Autodesk Fusion 360 part; units mm, degrees
(part 2 of 2)
sketch "Sketch26" plane through (0, 0, -29.65) normal (0, 0, 1) x (-1, 0, 0)
  circle A0 centre (-271.74, -5) radius 4.5
  circle A1 centre (-155, -82.8) radius 4.5
  circle A2 centre (-271.74, -82.8) radius 4.5
  circle A3 centre (-155, -5) radius 4.5
  line L0 (-186.5, -86) -> (-186.5, -90)
  line L1 (-186.5, -90) -> (-147, -90)
  line L2 (-147, -90) -> (-147, 7)
  line L3 (-147, 7) -> (-282, 7)
  line L4 (-282, 7) -> (-282, -90)
  line L5 (-282, -90) -> (-233, -90)
  line L6 (-233, -90) -> (-233, -86)
  line L7 (-233, -86) -> (-186.5, -86)
  line L8 (-243, -90) -> (-263, -90)
  line L9 (-263, -90) -> (-263, -72)
  line L10 (-263, -72) -> (-243, -72)
  line L11 (-243, -72) -> (-243, -90)
  dimension "d246" = 20
  dimension "d247" = 10
  dimension "d248" = 18
  constraint horizontal L8
  constraint vertical L9
  constraint horizontal L10
  constraint vertical L11
  constraint coincident L5 L8.start
  measures "d246" distance of L9 L11
  measures "d247" distance of L6 L11
  measures "d248" distance of L8.end L9.end
extrude "Extrude25" add sketch "Sketch26" along normal blind 5 contours L5 L8 L9 L10 L11 bodies 34
sketch "Sketch27" plane through (0, 0, -24.65) normal (0, 0, 1) x (-1, 0, 0)
  line L0 (-243, -72) -> (-263, -72)
  line L1 (-263, -72) -> (-263, -90)
  line L2 (-263, -90) -> (-243, -90)
  line L3 (-243, -90) -> (-243, -72)
  line L4 (-243, -90) -> (-243.9, -90)
  line L5 (-243.9, -90) -> (-243.9, -72)
  line L6 (-243.9, -72) -> (-243, -72)
  line L7 (-243, -72) -> (-243, -90)
  line L8 (-243.9, -72) -> (-263, -72)
  line L9 (-263, -72) -> (-263, -72.9)
  line L10 (-263, -72.9) -> (-243.9, -72.9)
  line L11 (-243.9, -72.9) -> (-243.9, -72)
  line L12 (-263, -72.9) -> (-262.1, -72.9)
  line L13 (-262.1, -72.9) -> (-262.1, -90)
  line L14 (-262.1, -90) -> (-263, -90)
  line L15 (-263, -90) -> (-263, -72.9)
  dimension "d251" = 0.9
  dimension "d252" = 0.9
  dimension "d253" = 0.9
  constraint horizontal L4
  constraint vertical L5
  constraint horizontal L6
  constraint vertical L7
  constraint coincident L0 L5.end
  constraint coincident L2.end L3.start
  constraint horizontal L8
  constraint vertical L9
  constraint horizontal L10
  constraint vertical L11
  constraint coincident L1 L9.end
  constraint horizontal L12
  constraint vertical L13
  constraint horizontal L14
  constraint vertical L15
  constraint coincident L2 L13.end
  measures "d251" distance of L8 L10
  measures "d252" distance of L5 L7
  measures "d253" distance of L13 L15
extrude "Extrude26" add sketch "Sketch27" along normal blind 1 contours L0 L2 L3 L4 L5 L6 L7 L11 | L0 L1 L5 L8 L9 L10 L11 L12 | L1 L2 L10 L12 L13 L14 L15 bodies 34
sketch "Sketch29" plane through (0, 90, 0) normal (0, -1, 0) x (1, 0, 0)
  line L0 (243, -29.65) -> (243, -23.65)
  line L1 (243, -23.65) -> (243.9, -23.65)
  line L2 (243.9, -23.65) -> (243.9, -24.65)
  line L3 (243.9, -24.65) -> (262.1, -24.65)
  line L4 (262.1, -24.65) -> (262.1, -23.65)
  line L5 (262.1, -23.65) -> (263, -23.65)
  line L6 (263, -23.65) -> (263, -29.65)
  line L7 (263, -29.65) -> (282, -29.65)
  line L8 (282, -29.65) -> (282, -12.65)
  line L9 (282, -12.65) -> (233, -12.65)
  line L10 (233, -12.65) -> (233, -29.65)
  line L11 (233, -29.65) -> (243, -29.65)
  line L12 (248.95, -21) -> (257.3, -21)
  line L13 (257.3, -21) -> (257.3, -25.6)
  line L14 (257.3, -25.6) -> (248.95, -25.6)
  line L15 (248.95, -25.6) -> (248.95, -21)
  dimension "d256" = 5.05
  dimension "d257" = 8.35
  dimension "d258" = 4.6
  dimension "d259" = 3.65
  constraint horizontal L12
  constraint vertical L13
  constraint horizontal L14
  constraint vertical L15
  measures "d256" horizontal distance of L2.end L14.end
  measures "d257" distance of L12.start L12.end
  measures "d258" distance of L12.end L13.end
  measures "d259" distance of L3 L12
extrude "Extrude27" cut sketch "Sketch29" along normal blind -3 and the other way blind -3 contours L3 L12 L13 L15 | L3 L13 L14 L15 bodies 34
sketch "Sketch30" plane through (0, 0, -24.65) normal (0, 0, 1) x (-1, 0, 0)
  line L0 (-248.95, -87) -> (-248.95, -90)
  line L1 (-248.95, -90) -> (-243.9, -90)
  line L2 (-243.9, -90) -> (-243.9, -72.9)
  line L3 (-243.9, -72.9) -> (-262.1, -72.9)
  line L4 (-262.1, -72.9) -> (-262.1, -90)
  line L5 (-262.1, -90) -> (-257.3, -90)
  line L6 (-257.3, -90) -> (-257.3, -87)
  line L7 (-257.3, -87) -> (-248.95, -87)
  circle A0 centre (-247.95, -79.45) radius 1
  circle A1 centre (-258.05, -79.45) radius 1
  dimension "d264" = 4.05
  dimension "d265" = 4.05
  dimension "d266" = 6.55
  dimension "d267" = 6.55
  dimension "d268" = 2
  dimension "d269" = 2
  measures "d264" distance of L2 A0.centre
  measures "d265" distance of L4 A1.centre
  measures "d266" distance of L3 A1.centre
  measures "d267" distance of L3 A0.centre
  measures "d268" diameter of A0
  measures "d269" diameter of A1
extrude "Extrude28" cut sketch "Sketch30" against normal blind 5 contours A0 | A1 bodies 34
sketch "Sketch32" plane through (0, 0, -10) normal (0, 0, 1) x (-1, 0, 0)
  line L0 (-155, -1.5359) -> (-152, -3.2679)
  line L1 (-152, -3.2679) -> (-152, -6.7321)
  line L2 (-152, -6.7321) -> (-155, -8.4641)
  line L3 (-155, -8.4641) -> (-158, -6.7321)
  line L4 (-158, -6.7321) -> (-158, -3.2679)
  line L5 (-158, -3.2679) -> (-155, -1.5359)
  circle A0 centre (-155, -5) radius 4.5
  circle A1 centre (-155, -5) radius 2
  circle A2 centre (-155, -82.8) radius 2
  circle A3 centre (-271.74, -82.8) radius 2
  circle A4 centre (-271.74, -5) radius 2
  circle A5 centre (-271.74, -5) radius 4.5
  circle A6 centre (-271.74, -82.8) radius 4.5
  circle A7 centre (-155, -82.8) radius 4.5
  dimension "d272" = 4
  dimension "d273" = 4
  dimension "d274" = 4
  dimension "d275" = 4
  constraint concentric A0 A1
  constraint concentric A4 A5
  constraint concentric A3 A6
  constraint concentric A2 A7
  measures "d272" diameter of A1
  measures "d273" diameter of A2
  measures "d274" diameter of A3
  measures "d275" diameter of A4
extrude "Extrude29" cut sketch "Sketch32" against normal through all contours A1 | A2 | A3 | A4 bodies 34
sketch "Sketch33" plane through (0, 0, -32.65) normal (0, 0, -1) x (1, 0, 0)
  circle A0 centre (155, -5) radius 2
  circle A1 centre (271.74, -5) radius 2
  circle A2 centre (155, -82.8) radius 2
  circle A3 centre (271.74, -82.8) radius 2
  line L0 (290, -83) -> (285, -83)
  line L1 (285, -83) -> (285, 42)
  line L2 (285, 42) -> (290, 42)
  line L3 (290, 42) -> (290, -83)
  line L4 (295, -88) -> (295, 47)
  arc A4 (295, 47) -> (290, 52) centre (290, 47) ccw
  line L5 (290, 52) -> (139, 52)
  arc A5 (139, 52) -> (134, 47) centre (139, 47) ccw
  line L6 (134, 47) -> (134, -88)
  arc A6 (134, -88) -> (139, -93) centre (139, -88) ccw
  line L7 (139, -93) -> (290, -93)
  arc A7 (290, -93) -> (295, -88) centre (290, -88) ccw
  line L8 (139, -83) -> (139, 42)
  line L9 (139, 42) -> (144, 42)
  line L10 (144, 42) -> (144, -83)
  line L11 (144, -83) -> (139, -83)
  circle A8 centre (155, -5) radius 4.5
  circle A9 centre (271.74, -5) radius 4.5
  circle A10 centre (155, -82.8) radius 4.5
  circle A11 centre (271.74, -82.8) radius 4.5
  dimension "d277" = 9
  dimension "d278" = 9
  dimension "d279" = 9
  dimension "d280" = 9
  constraint concentric A0 A8
  constraint concentric A1 A9
  constraint concentric A2 A10
  constraint concentric A3 A11
  measures "d277" diameter of A8
  measures "d278" diameter of A9
  measures "d279" diameter of A10
  measures "d280" diameter of A11
extrude "Extrude30" cut sketch "Sketch33" against normal blind 1 contours A8 | A9 | A10 | A11 bodies 34
move_body "Move19" bodies 36 to x (1, 0, 0) y (0, 1, 0) z (0, 0, 1) at (0, 57, 0)
move_body "Move20" bodies 36 to x (1, 0, 0) y (0, 1, 0) z (0, 0, 1) at (0.2606, 11.9381, -1)
combine "Combine1" operation add target body 35 tool bodies 36
move_body "Move21" bodies 34 to x (1, 0, 0) y (0, 1, 0) z (0, 0, 1) at (-170, 0, 0)
sketch "Sketch34" plane through (0, -52, 0) normal (0, -1, 0) x (1, 0, 0)
  line L0 (115, 16.35) -> (-26, 16.35)
  line L1 (-26, 16.35) -> (-26, 6.35)
  line L2 (-26, 6.35) -> (-31, 6.35)
  line L3 (-31, 6.35) -> (-31, -12.65)
  line L4 (-31, -12.65) -> (120, -12.65)
  line L5 (120, -12.65) -> (120, 6.35)
  line L6 (120, 6.35) -> (115, 6.35)
  line L7 (115, 6.35) -> (115, 16.35)
  circle A0 centre (105.1711, 6.35) radius 6
  circle A1 centre (105.1711, -21.65) radius 6
  line L8 (120, -32.65) -> (-31, -32.65)
  dimension "d286" = 12
  dimension "d287" = 10
  dimension "d288" = 12
  dimension "d289" = 11
  constraint vertical A0.centre A1.centre
  measures "d286" diameter of A0
  measures "d287" distance of L0 A0.centre
  measures "d288" diameter of A1
  measures "d289" distance of A1.centre L8
extrude "Extrude31" cut sketch "Sketch34" against normal blind 3 contours A1 bodies 34
extrude "Extrude32" cut sketch "Sketch34" against normal blind 3 contours A0 bodies 35
sketch "Sketch35" plane through (0, -7, 0) normal (0, 1, 0) x (-1, 0, 0)
  line L0 (-112, -12.65) -> (23, -12.65)
  line L1 (23, -12.65) -> (23, 13.35)
  line L2 (23, 13.35) -> (-112, 13.35)
  line L3 (-112, 13.35) -> (-112, -12.65)
  line L4 (-102, 6.35) -> (-37, 6.35)
  line L5 (-37, 6.35) -> (-37, -21.65)
  line L6 (-37, -21.65) -> (-102, -21.65)
  line L7 (-102, -21.65) -> (-102, 6.35)
  line L8 (23, -29.65) -> (-112, -29.65)
  dimension "d294" = 8
  dimension "d295" = 7
  dimension "d296" = 10
  dimension "d297" = 60
  dimension "d298" = 43
  constraint horizontal L4
  constraint vertical L5
  constraint horizontal L6
  constraint vertical L7
  measures "d294" distance of L6 L8
  measures "d295" distance of L2 L4
  measures "d296" distance of L3 L7
  measures "d297" distance of L1 L5
  measures "d298" distance of L2 L8
extrude "Extrude33" cut sketch "Sketch35" against normal blind 3 contours L0 L4 L5 L7 | L0 L5 L6 L7 bodies 34 35
sketch "Sketch36" plane through (0, 0, -10) normal (0, 0, 1) x (-1, 0, 0)
  line L0 (-101.74, -1.5359) -> (-98.74, -3.2679)
  line L1 (-98.74, -3.2679) -> (-98.74, -6.7321)
  line L2 (-98.74, -6.7321) -> (-101.74, -8.4641)
  line L3 (-101.74, -8.4641) -> (-104.74, -6.7321)
  line L4 (-104.74, -6.7321) -> (-104.74, -3.2679)
  line L5 (-104.74, -3.2679) -> (-101.74, -1.5359)
  circle A0 centre (-101.74, -5) radius 4.5
  line L6 (-101.74, -5) -> (-114.9756, -5) construction
  constraint coincident A0.centre L6.start
  constraint perpendicular L4 L6
sketch "Sketch37" plane through (112, 0, 0) normal (-1, 0, 0) x (0, -1, 0)
  line L0 (-90, -12.65) -> (7, -12.65)
  line L1 (7, -12.65) -> (7, 13.35)
  line L2 (7, 13.35) -> (-90, 13.35)
  line L3 (-90, 13.35) -> (-90, -12.65)
  line L4 (-4.9879, -9.9902) -> (-16.9879, -9.9902) construction
  line L5 (-16.9879, -12.65) -> (-29.3879, -12.65)
  line L6 (-29.3879, -12.65) -> (-29.3879, -6.9)
  line L7 (-29.3879, -6.9) -> (-16.9879, -6.9)
  line L8 (-16.9879, -6.9) -> (-16.9879, -12.65)
  line L9 (-29.3879, -12.65) -> (-16.9879, -12.65)
  line L10 (-16.9879, -12.65) -> (-16.9879, -18.4)
  line L11 (-16.9879, -18.4) -> (-29.3879, -18.4)
  line L12 (-29.3879, -18.4) -> (-29.3879, -12.65)
  dimension "d301" = 12
  dimension "d302" = 12.4
  dimension "d303" = 5.75
  dimension "d304" = 12.4
  dimension "d305" = 5.75
  constraint parallel L0 L4
  constraint horizontal L5
  constraint vertical L6
  constraint horizontal L7
  constraint vertical L8
  constraint coincident L0 L5.start
  constraint coincident L4.end L8
  constraint horizontal L9
  constraint vertical L10
  constraint horizontal L11
  constraint vertical L12
  measures "d301" distance of L4.start L4.end
  measures "d302" distance of L5.start L5.end
  measures "d303" distance of L5.start L7.end
  measures "d304" distance of L5.end L5.start
  measures "d305" distance of L5.end L11.end
extrude "Extrude34" cut sketch "Sketch37" against normal blind 3 contours L0 L5 L6 L7 L8 L9 | L0 L5 L9 L10 L11 L12 bodies 34 35
move_body "Move22" bodies 35 to x (1, 0, 0) y (0, 1, 0) z (0, 0, 1) at (190, 0, 0)
move_body "Move23" bodies 35 to x (-1, 0, 0) y (0, 1, 0) z (0, 0, -1) at (358, 0, 32.7)
move_body "Move24" bodies 35 to x (1, 0, 0) y (0, 1, 0) z (0, 0, 1) at (110, 0, -50)
move_body "Move25" bodies 35 to x (1, 0, 0) y (0, 1, 0) z (0, 0, 1) at (0, 0, 30)
move_body "Move26" bodies 34 to x (1, 0, 0) y (0, 1, 0) z (0, 0, 1) at (0, 0, 30)
sketch "Sketch38" plane through (0, 0, -3.65) normal (0, 0, -1) x (1, 0, 0)
  line L0 (180, -83.5) -> (180, -32.5)
  arc A0 (185, -27.5) -> (180, -32.5) centre (185, -32.5) ccw
  line L1 (185, -27.5) -> (284, -27.5)
  arc A1 (289, -32.5) -> (284, -27.5) centre (284, -32.5) ccw
  line L2 (289, -32.5) -> (289, -83.5)
  arc A2 (284, -88.5) -> (289, -83.5) centre (284, -83.5) ccw
  line L3 (284, -88.5) -> (185, -88.5)
  arc A3 (180, -83.5) -> (185, -88.5) centre (185, -83.5) ccw
  line L4 (304, 52) -> (163, 52)
  line L5 (163, 52) -> (163, -93)
  line L6 (163, -93) -> (304, -93)
  line L7 (304, -93) -> (304, 52)
  line L8 (304, 52) -> (163, 52) construction
  line L9 (163, 52) -> (163, -4.5554) construction
  line L10 (163, -4.5554) -> (304, -4.5554) construction
  line L11 (304, -4.5554) -> (304, 52) construction
  line L12 (304, 31.5751) -> (163, 31.5751) construction
  line L13 (163, 31.5751) -> (163, -27.5) construction
  line L14 (163, -27.5) -> (304, -27.5) construction
  line L15 (304, -27.5) -> (304, 31.5751) construction
  dimension "d309" = 12
  dimension "d314" = 16
  text T0 "IF4Health" font "Arial Black" height 12 align centre middle in box 141 x 56.5554 at (304, 52) x (-1, 0) y (0, -1) spacing 1 kerned
  text T1 "BIoT" font "Arial Black" height 16 align centre middle in box 141 x 59.0751 at (304, 31.5751) x (-1, 0) y (0, -1) spacing 1 kerned
  constraint coincident L5
  constraint coincident L4.start
  constraint coincident L4
  constraint coincident L7
extrude "Extrude35" cut sketch "Sketch38" against normal blind 1 text T0 bodies 35
extrude "Extrude36" cut sketch "Sketch38" against normal blind 1 text T1 bodies 35
sketch "Sketch42" plane through (0, 0, 25.35) normal (0, 0, 1) x (-1, 0, 0)
  line L0 (-166, -16.9879) -> (-163, -16.9879)
  line L1 (-163, -16.9879) -> (-163, 42)
  line L2 (-163, 42) -> (-158, 42)
  arc A0 (-158, 42) -> (-158, 52) centre (-158, 47) ccw
  line L3 (-158, 52) -> (-309, 52)
  arc A1 (-309, 52) -> (-309, 42) centre (-309, 47) ccw
  line L4 (-309, 42) -> (-304, 42)
  line L5 (-304, 42) -> (-304, -83)
  line L6 (-304, -83) -> (-309, -83)
  arc A2 (-309, -83) -> (-309, -93) centre (-309, -88) ccw
  line L7 (-309, -93) -> (-158, -93)
  arc A3 (-158, -93) -> (-158, -83) centre (-158, -88) ccw
  line L8 (-158, -83) -> (-163, -83)
  line L9 (-163, -83) -> (-163, -29.3879)
  line L10 (-163, -29.3879) -> (-166, -29.3879)
  line L11 (-166, -29.3879) -> (-166, -90)
  line L12 (-166, -90) -> (-301, -90)
  line L13 (-301, -90) -> (-301, 7)
  line L14 (-301, 7) -> (-241, 7)
  line L15 (-241, 7) -> (-241, 10)
  line L16 (-241, 10) -> (-301, 10)
  line L17 (-301, 10) -> (-301, 49)
  line L18 (-301, 49) -> (-166, 49)
  line L19 (-166, 49) -> (-166, 10)
  line L20 (-166, 10) -> (-176, 10)
  line L21 (-176, 10) -> (-176, 7)
  line L22 (-176, 7) -> (-166, 7)
  line L23 (-166, 7) -> (-166, -16.9879)
  line L24 (-241, 7) -> (-261, 7)
  line L25 (-261, 7) -> (-261, 10)
  dimension "d317" = 20
  constraint coincident L14.end L15.start
  constraint perpendicular L15 L24
  constraint coincident L16 L25.end
  constraint perpendicular L16 L25
  measures "d317" distance of L14.end L24.end
extrude "Extrude37" cut sketch "Sketch42" against normal up to surface (19 mm away) contours L14 L15 L16 L24 L25 bodies 35
component "Component" placed x (1, 0, 0) y (0, 1, 0) z (0, 0, 1) at (0, 0, 0)
component "Component'" placed x (1, 0, 0) y (0, 1, 0) z (0, 0, 1) at (0, 0, 0)
component "Component''" placed x (1, 0, 0) y (0, 1, 0) z (0, 0, 1) at (0, 0, 0)
component "Component'''" placed x (1, 0, 0) y (0, 1, 0) z (0, 0, 1) at (0, 0, 0)
component "Component''''" placed x (1, 0, 0) y (0, 1, 0) z (0, 0, 1) at (0, 0, 0)
component "Component'''''" placed x (1, 0, 0) y (0, 1, 0) z (0, 0, 1) at (0, 0, 0)
component "Component''''''" placed x (1, 0, 0) y (0, 1, 0) z (0, 0, 1) at (0, 0, 0)
component "Component'''''''" placed x (1, 0, 0) y (0, 1, 0) z (0, 0, 1) at (0, 0, 0)
component "Component''''''''" placed x (1, 0, 0) y (0, 1, 0) z (0, 0, 1) at (0, 0, 0)
component "Component'''''''''" placed x (1, 0, 0) y (0, 1, 0) z (0, 0, 1) at (0, 0, 0)
component "Component''''''''''" placed x (1, 0, 0) y (0, 1, 0) z (0, 0, 1) at (0, 0, 0)
component "Component'''''''''''" placed x (1, 0, 0) y (0, 1, 0) z (0, 0, 1) at (0, 0, 0)
hidden bodies 1 10 11 12 13 33
equation "d117 = ( 14.25 / 2 ) * 1 mm"
